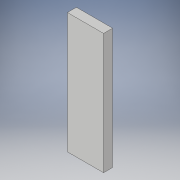
# Autodesk Inventor part: double door
Saved by Autodesk Inventor 2017 (Build 210142000, 142)
## iProperties
Created: 2018-03-03
Part Number: double door
Material: Generic
Document SubType Name: Modeling
Designer: Braxton
Density: 1 g/cm^3
Appearance: Default
Author: Braxton
Autodesk Inventor part; units mm, degrees
ref_plane "YZ Plane" through (0, 0, 0) normal (1, 0, 0) x (0, 1, 0)
ref_plane "XZ Plane" through (0, 0, 0) normal (0, 1, 0) x (-1, 0, 0)
ref_plane "XY Plane" through (0, 0, 0) normal (0, 0, 1) x (1, 0, 0)
sketch "Sketch1" plane through (0, 0, 0) normal (0, 0, 1) x (1, 0, 0)
  line L0 (0, 0) -> (50.8, 0)
  line L1 (50.8, 0) -> (50.8, 169.3333)
  line L2 (50.8, 169.3333) -> (0, 169.3333)
  line L3 (0, 169.3333) -> (0, 0)
  dimension "d0" = 50.8
  dimension "d1" = 169.3333
  constraints: 8 end point, 3 perpendicular, 1 horizontal
  measures "d0" distance of L0.start L0.end
  measures "d1" distance of L0.end L1.end
extrude "door half" add sketch "Sketch1" along normal blind 12.7
body "Solid1"
